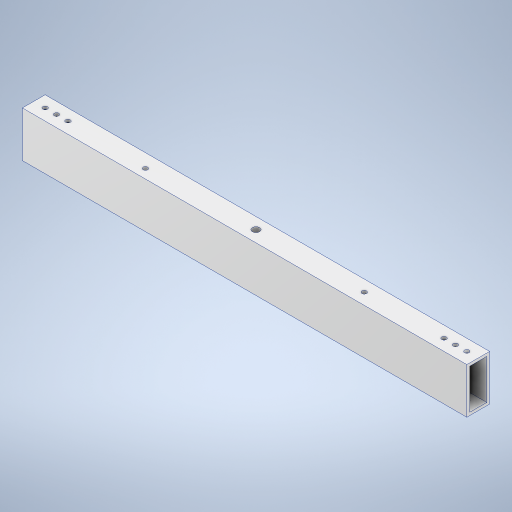
# Autodesk Inventor part: (b)swerveassembly
Saved by Autodesk Inventor 2024 (Build 280153000, 153)
## iProperties
Created: 2023-09-27
Part Number: (b)swerveassembly
Material: Aluminum 6061
Document SubType Name: Modeling
Designer: s137416
Density: 2.7 g/cm^3
Appearance: Aluminum - Flat
Author: s137416
Autodesk Inventor part; units mm, degrees
ref_plane "YZ Plane" through (0, 0, 0) normal (1, 0, 0) x (0, 1, 0)
ref_plane "XZ Plane" through (0, 0, 0) normal (0, 1, 0) x (-1, 0, 0)
ref_plane "XY Plane" through (0, 0, 0) normal (0, 0, 1) x (1, 0, 0)
sketch "Sketch1" plane through (0, 0, 0) normal (0, 0, 1) x (1, 0, 0)
  line L0 (-187.4297, 132.1193) -> (307.8703, 132.1193)
  line L1 (307.8703, 132.1193) -> (307.8703, 81.3193)
  line L2 (307.8703, 81.3193) -> (-187.4297, 81.3193)
  line L3 (-187.4297, 81.3193) -> (-187.4297, 132.1193)
  point P0 (0, 0)
  dimension "d0" = 495.3
  dimension "d1" = 50.8
  constraints: 8 end point, 2 parallel, 1 horizontal, 1 perpendicular
  measures "d0" distance of L0.start L0.end
  measures "d1" distance of L2.end L0.start
extrude "Extrusion1" add sketch "Sketch1" along normal blind 25.4
sketch "Sketch2" plane through (-187.4297, 132.1193, 0) normal (0, 1, 0) x (1, 0, 0)
  circle A0 centre (12.7, -12.7) radius 2.5019
  line L0 (0, 0) -> (0, -25.4) projected
  circle A1 centre (25.4, -12.7) radius 2.5019
  circle A2 centre (38.1, -12.7) radius 2.5019
  circle A3 centre (482.6, -12.7) radius 2.5019
  line L1 (495.3, 0) -> (495.3, -25.4) projected
  circle A4 centre (469.9, -12.7) radius 2.5019
  circle A5 centre (457.2, -12.7) radius 2.5019
  circle A6 centre (368.3, -12.7) radius 2.5527
  circle A7 centre (127, -15.2019) radius 2.5527
  circle A8 centre (247.65, -12.7) radius 3.9751
  line L2 (495.3, 0) -> (0, 0) projected
  point P0 (187.4297, 0)
  dimension "d4" = 12.7
  dimension "d5" = 5.0038
  dimension "d6" = 5.0038
  dimension "d7" = 5.0038
  dimension "d8" = 12.7
  dimension "d9" = 12.7
  dimension "d10" = 5.0038
  dimension "d11" = 12.7
  dimension "d12" = 5.0038
  dimension "d13" = 5.0038
  dimension "d14" = 12.7
  dimension "d15" = 12.7
  dimension "d19" = 127
  dimension "d20" = 5.1054
  dimension "d21" = 5.1054
  dimension "d22" = 127
  dimension "d23" = 7.9502
  dimension "d24" = 247.65
  dimension "d25" = 12.7
  constraints: 9 centre point
  measures "d4" distance from line of L0 A0.centre
  measures "d5" diameter of A0
  measures "d6" diameter of A1
  measures "d7" diameter of A2
  measures "d8" distance of A0.centre A1.centre
  measures "d9" distance of A1.centre A2.centre
  measures "d10" diameter of A3
  measures "d11" distance from line of L1 A3.centre
  measures "d12" diameter of A5
  measures "d13" diameter of A4
  measures "d14" distance of A3.centre A4.centre
  measures "d15" distance of A5.centre A4.centre
  measures "d19" distance from line of L1 A6.centre
  measures "d20" diameter of A6
  measures "d21" diameter of A7
  measures "d22" distance from line of L0 A7.centre
  measures "d23" diameter of A8
  measures "d24" distance from line of L0 A8.centre
  measures "d25" distance from line of L2 A8.centre
extrude "Extrusion2" cut sketch "Sketch2" against normal blind 50.8
shell "Shell1" thickness 3.175 removed faces 8 at (307.8703, 98.2527, 8.4667) at (295.0696, 98.2527, 10.2001) at (269.6696, 98.2527, 10.2001) at (282.3696, 98.2527, 10.2001) at (-187.4297, 115.186, 16.9333) at (-174.8304, 98.2527, 10.2001) at (-149.4304, 98.2527, 10.2001) at (-162.1304, 98.2527, 10.2001)
body "Solid1"
